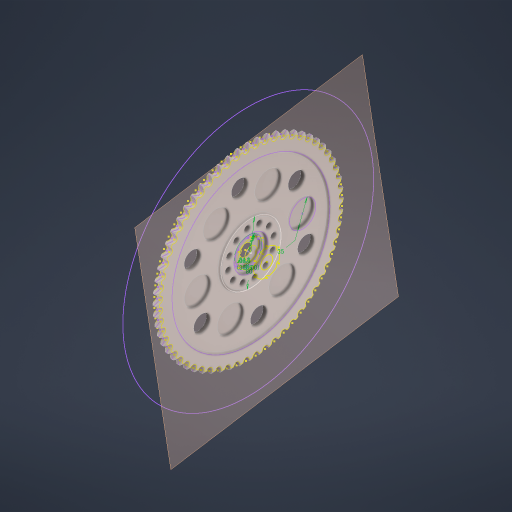
# Autodesk Inventor part: 40A60_()
Saved by Autodesk Inventor 2024.3 (Build 283343000, 343)
## iProperties
Category: PARTsolutions
Company: KANA
Created: 2025-03-03
Part Number: 40A60_()
Material: Generic
Catalog Web Link: www.cadenas.de
Description: 40A-Un-finished
Vendor: KANA
Document SubType Name: Modeling
Designer: psAdmin
Manufacturer: KANA
Mass: 324.137 g
Surface Area: 991.07 cm^2
Volume: 324.137 cm^3
Density: 1 g/cm^3
Appearance: PSOLRGB-175-175-175
PSOL_IDENT_0: {$CADENAS_DATA/23d-libs/kana/sprockets/chain_no_40/un_finished_sprcoket_steel/a_type/40a.prj},156 {V
PSOL_IDENT_1: TYP=3D},{NB=40A60_()},{LINA=40A60},{NN=40A},{DATE=27.06.2023 01:46:20},{GEOMDATE=02.10.2020 05:05:43
PSOL_IDENT_2: },{VERSION=},{LINEID=490},{WBVAR=SURFT},{WBNUMERIC=}  {NB=40A60_()},{LINA=40A60},{KT=DUMMY},{ORDERNO=
PSOL_IDENT_3: 40A60},{TYPE=40A},{NOT=60},{NOTX=60.000},{DP=242.66},{DC=234.71},{DC2=234.71},{DO=250},{T=7.2},{DR=7
PSOL_IDENT_4: .950},{MAT=None},{MATC=},{SD=16},{SURFT=},{SURFTNB=},{DCX2=0},{CAUTION=The tooth profile in the CAD
PSOL_IDENT_5: models differ from the actual shape.}
NB: 40A60_()
NN: 40A
NT: Un-finished
NBSYN: 40A$NOT._($SURFT.)
LINA: 40A60
CATALOG: KANA
TYPE: 40A
NOT: 60
DP: 242.66
DC: 234.71
DC2: 234.71
DO: 250
T: 7.2
SD: 16
SURFT: No symbol : No
CAUTION: The tooth profile in the CAD models differ from the actual shape.
SUPPLIER: KANA
ARTICLENO: 40A60_()
BOMINFO: 40A60
CREATOR: CADENAS GmbH
Title: 40A60
Author: Cadenas PARTsolutions
Comments: Un-finished
Autodesk Inventor part; units mm, degrees
(part 1 of 2)
ref_plane "YZ Plane" through (0, 0, 0) normal (1, 0, 0) x (0, 1, 0)
ref_plane "XZ Plane" through (0, 0, 0) normal (0, 1, 0) x (-1, 0, 0)
ref_plane "XY Plane" through (0, 0, 0) normal (0, 0, 1) x (1, 0, 0)
sketch "Sketch_1" plane through (0, 0, 0) normal (0, 0, 1) x (1, 0, 0)
  line L0 (7.2, 0) -> (0, 0)
  line L1 (0, 8) -> (7.2, 8)
  line L2 (7.2, 8) -> (7.2, 121.6682)
  arc A0 (7.2, 121.6682) -> (5.4, 125) centre (-0.4933, 119.6641) ccw
  line L3 (5.4, 125) -> (1.8, 125)
  arc A1 (1.8, 125) -> (0, 121.6682) centre (7.6933, 119.6641) ccw
  line L4 (0, 121.6682) -> (0, 8)
  constraints: 10 end point, 4 point on circle, 2 centre point
revolve "Revolution1" add sketch "Sketch_1" angle 360 about axis through (7.2, 0, 0) along (1, 0, 0)
sketch "Sketch_2" plane through (3.6, 0, 0) normal (1, 0, 0) x (0, 0, -1)
  circle A0 centre (0, 0) radius 166.6667
  arc A1 (-124.999, 0.5) -> (-124.999, -0.5) centre (0, 0) ccw
  line L0 (-124.999, -0.5) -> (-119.6668, -2.6675)
  arc A2 (-119.2901, -9.8557) -> (-119.6668, -2.6675) centre (-121.1637, -6.3499) ccw
  line L1 (-119.2901, -9.8557) -> (-124.3665, -12.5687)
  arc A3 (-124.3665, -12.5687) -> (-124.262, -13.5632) centre (0, 0) ccw
  line L2 (-124.262, -13.5632) -> (-118.7324, -15.1615)
  arc A4 (-117.6064, -22.2709) -> (-118.7324, -15.1615) centre (-119.8362, -18.9802) ccw
  line L3 (-117.6064, -22.2709) -> (-122.3714, -25.4997)
  arc A5 (-122.3714, -25.4997) -> (-122.1635, -26.4778) centre (0, 0) ccw
  line L4 (-122.1635, -26.4778) -> (-116.4972, -27.4894)
  arc A6 (-114.6342, -34.4421) -> (-116.4972, -27.4894) centre (-117.1958, -31.4025) ccw
  line L5 (-114.6342, -34.4421) -> (-119.0356, -38.1513)
  arc A7 (-119.0356, -38.1513) -> (-118.7266, -39.1023) centre (0, 0) ccw
  line L6 (-118.7266, -39.1023) -> (-112.9856, -39.5161)
  arc A8 (-110.4061, -46.236) -> (-112.9856, -39.5161) centre (-113.2713, -43.4808) ccw
  line L7 (-110.4061, -46.236) -> (-114.3956, -50.3849)
  arc A9 (-114.3956, -50.3849) -> (-113.9889, -51.2984) centre (0, 0) ccw
  line L8 (-113.9889, -51.2984) -> (-108.2361, -51.1098)
  arc A10 (-104.9683, -57.5233) -> (-108.2361, -51.1098) centre (-108.1058, -55.0827) ccw
  line L9 (-104.9683, -57.5233) -> (-108.5023, -62.0665)
  arc A11 (-108.5023, -62.0665) -> (-108.0023, -62.9325) centre (0, 0) ccw
  line L10 (-108.0023, -62.9325) -> (-102.3007, -62.1436)
  arc A12 (-98.3804, -68.1803) -> (-102.3007, -62.1436) centre (-101.7559, -66.0811) ccw
  line L11 (-98.3804, -68.1803) -> (-101.4202, -73.0681)
  arc A13 (-101.4202, -73.0681) -> (-100.8324, -73.8771) centre (0, 0) ccw
  line L12 (-100.8324, -73.8771) -> (-95.2446, -72.4965)
  arc A14 (-90.7147, -78.0904) -> (-95.2446, -72.4965) centre (-94.2911, -76.3554) ccw
  line L13 (-90.7147, -78.0904) -> (-93.2269, -83.2691)
  arc A15 (-93.2269, -83.2691) -> (-92.5578, -84.0122) centre (0, 0) ccw
  line L14 (-92.5578, -84.0122) -> (-87.1448, -82.0551)
  arc A16 (-82.0551, -87.1448) -> (-87.1448, -82.0551) centre (-85.7933, -85.7933) ccw
  line L15 (-82.0551, -87.1448) -> (-84.0122, -92.5578)
  arc A17 (-84.0122, -92.5578) -> (-83.2691, -93.2269) centre (0, 0) ccw
  line L16 (-83.2691, -93.2269) -> (-78.0904, -90.7147)
  arc A18 (-72.4965, -95.2446) -> (-78.0904, -90.7147) centre (-76.3554, -94.2911) ccw
  line L17 (-72.4965, -95.2446) -> (-73.8771, -100.8324)
  arc A19 (-73.8771, -100.8324) -> (-73.0681, -101.4202) centre (0, 0) ccw
  line L18 (-73.0681, -101.4202) -> (-68.1803, -98.3804)
  arc A20 (-62.1436, -102.3007) -> (-68.1803, -98.3804) centre (-66.0811, -101.7559) ccw
  line L19 (-62.1436, -102.3007) -> (-62.9325, -108.0023)
  arc A21 (-62.9325, -108.0023) -> (-62.0665, -108.5023) centre (0, 0) ccw
  line L20 (-62.0665, -108.5023) -> (-57.5233, -104.9683)
  arc A22 (-51.1098, -108.2361) -> (-57.5233, -104.9683) centre (-55.0827, -108.1058) ccw
  line L21 (-51.1098, -108.2361) -> (-51.2984, -113.9889)
  arc A23 (-51.2984, -113.9889) -> (-50.3849, -114.3956) centre (0, 0) ccw
  line L22 (-50.3849, -114.3956) -> (-46.236, -110.4061)
  arc A24 (-39.5161, -112.9856) -> (-46.236, -110.4061) centre (-43.4808, -113.2713) ccw
  line L23 (-39.5161, -112.9856) -> (-39.1023, -118.7266)
  arc A25 (-39.1023, -118.7266) -> (-38.1513, -119.0356) centre (0, 0) ccw
  line L24 (-38.1513, -119.0356) -> (-34.4421, -114.6342)
  arc A26 (-27.4894, -116.4972) -> (-34.4421, -114.6342) centre (-31.4025, -117.1958) ccw
  line L25 (-27.4894, -116.4972) -> (-26.4778, -122.1635)
  arc A27 (-26.4778, -122.1635) -> (-25.4997, -122.3714) centre (0, 0) ccw
  line L26 (-25.4997, -122.3714) -> (-22.2709, -117.6064)
  arc A28 (-15.1615, -118.7324) -> (-22.2709, -117.6064) centre (-18.9802, -119.8362) ccw
  line L27 (-15.1615, -118.7324) -> (-13.5632, -124.262)
  arc A29 (-13.5632, -124.262) -> (-12.5687, -124.3665) centre (0, 0) ccw
  line L28 (-12.5687, -124.3665) -> (-9.8557, -119.2901)
  arc A30 (-2.6675, -119.6668) -> (-9.8557, -119.2901) centre (-6.3499, -121.1637) ccw
  line L29 (-2.6675, -119.6668) -> (-0.5, -124.999)
  arc A31 (-0.5, -124.999) -> (0.5, -124.999) centre (0, 0) ccw
  line L30 (0.5, -124.999) -> (2.6675, -119.6668)
  arc A32 (9.8557, -119.2901) -> (2.6675, -119.6668) centre (6.3499, -121.1637) ccw
  line L31 (9.8557, -119.2901) -> (12.5687, -124.3665)
  arc A33 (12.5687, -124.3665) -> (13.5632, -124.262) centre (0, 0) ccw
  line L32 (13.5632, -124.262) -> (15.1615, -118.7324)
  arc A34 (22.2709, -117.6064) -> (15.1615, -118.7324) centre (18.9802, -119.8362) ccw
  line L33 (22.2709, -117.6064) -> (25.4997, -122.3714)
  arc A35 (25.4997, -122.3714) -> (26.4778, -122.1635) centre (0, 0) ccw
  line L34 (26.4778, -122.1635) -> (27.4894, -116.4972)
  arc A36 (34.4421, -114.6342) -> (27.4894, -116.4972) centre (31.4025, -117.1958) ccw
  line L35 (34.4421, -114.6342) -> (38.1513, -119.0356)
  arc A37 (38.1513, -119.0356) -> (39.1023, -118.7266) centre (0, 0) ccw
  line L36 (39.1023, -118.7266) -> (39.5161, -112.9856)
  arc A38 (46.236, -110.4061) -> (39.5161, -112.9856) centre (43.4808, -113.2713) ccw
  line L37 (46.236, -110.4061) -> (50.3849, -114.3956)
  arc A39 (50.3849, -114.3956) -> (51.2984, -113.9889) centre (0, 0) ccw
  line L38 (51.2984, -113.9889) -> (51.1098, -108.2361)
  arc A40 (57.5233, -104.9683) -> (51.1098, -108.2361) centre (55.0827, -108.1058) ccw
  line L39 (57.5233, -104.9683) -> (62.0665, -108.5023)
  arc A41 (62.0665, -108.5023) -> (62.9325, -108.0023) centre (0, 0) ccw
  line L40 (62.9325, -108.0023) -> (62.1436, -102.3007)
  arc A42 (68.1803, -98.3804) -> (62.1436, -102.3007) centre (66.0811, -101.7559) ccw
  line L41 (68.1803, -98.3804) -> (73.0681, -101.4202)
  arc A43 (73.0681, -101.4202) -> (73.8771, -100.8324) centre (0, 0) ccw
  line L42 (73.8771, -100.8324) -> (72.4965, -95.2446)
  arc A44 (78.0904, -90.7147) -> (72.4965, -95.2446) centre (76.3554, -94.2911) ccw
  line L43 (78.0904, -90.7147) -> (83.2691, -93.2269)
  arc A45 (83.2691, -93.2269) -> (84.0122, -92.5578) centre (0, 0) ccw
  line L44 (84.0122, -92.5578) -> (82.0551, -87.1448)
  arc A46 (87.1448, -82.0551) -> (82.0551, -87.1448) centre (85.7933, -85.7933) ccw
  line L45 (87.1448, -82.0551) -> (92.5578, -84.0122)
  arc A47 (92.5578, -84.0122) -> (93.2269, -83.2691) centre (0, 0) ccw
  line L46 (93.2269, -83.2691) -> (90.7147, -78.0904)
  arc A48 (95.2446, -72.4965) -> (90.7147, -78.0904) centre (94.2911, -76.3554) ccw
  line L47 (95.2446, -72.4965) -> (100.8324, -73.8771)
  arc A49 (100.8324, -73.8771) -> (101.4202, -73.0681) centre (0, 0) ccw
  line L48 (101.4202, -73.0681) -> (98.3804, -68.1803)
  arc A50 (102.3007, -62.1436) -> (98.3804, -68.1803) centre (101.7559, -66.0811) ccw
  line L49 (102.3007, -62.1436) -> (108.0023, -62.9325)
  arc A51 (108.0023, -62.9325) -> (108.5023, -62.0665) centre (0, 0) ccw
  line L50 (108.5023, -62.0665) -> (104.9683, -57.5233)
  arc A52 (108.2361, -51.1098) -> (104.9683, -57.5233) centre (108.1058, -55.0827) ccw
  line L51 (108.2361, -51.1098) -> (113.9889, -51.2984)
  arc A53 (113.9889, -51.2984) -> (114.3956, -50.3849) centre (0, 0) ccw
  line L52 (114.3956, -50.3849) -> (110.4061, -46.236)
  arc A54 (112.9856, -39.5161) -> (110.4061, -46.236) centre (113.2713, -43.4808) ccw
  line L53 (112.9856, -39.5161) -> (118.7266, -39.1023)
  arc A55 (118.7266, -39.1023) -> (119.0356, -38.1513) centre (0, 0) ccw
  line L54 (119.0356, -38.1513) -> (114.6342, -34.4421)
  arc A56 (116.4972, -27.4894) -> (114.6342, -34.4421) centre (117.1958, -31.4025) ccw
  line L55 (116.4972, -27.4894) -> (122.1635, -26.4778)
  arc A57 (122.1635, -26.4778) -> (122.3714, -25.4997) centre (0, 0) ccw
  line L56 (122.3714, -25.4997) -> (117.6064, -22.2709)
  arc A58 (118.7324, -15.1615) -> (117.6064, -22.2709) centre (119.8362, -18.9802) ccw
  line L57 (118.7324, -15.1615) -> (124.262, -13.5632)
  arc A59 (124.262, -13.5632) -> (124.3665, -12.5687) centre (0, 0) ccw
  line L58 (124.3665, -12.5687) -> (119.2901, -9.8557)
  arc A60 (119.6668, -2.6675) -> (119.2901, -9.8557) centre (121.1637, -6.3499) ccw
  line L59 (119.6668, -2.6675) -> (124.999, -0.5)
  arc A61 (124.999, -0.5) -> (124.999, 0.5) centre (0, 0) ccw
  line L60 (124.999, 0.5) -> (119.6668, 2.6675)
  arc A62 (119.2901, 9.8557) -> (119.6668, 2.6675) centre (121.1637, 6.3499) ccw
  line L61 (119.2901, 9.8557) -> (124.3665, 12.5687)
  arc A63 (124.3665, 12.5687) -> (124.262, 13.5632) centre (0, 0) ccw
  line L62 (124.262, 13.5632) -> (118.7324, 15.1615)
  arc A64 (117.6064, 22.2709) -> (118.7324, 15.1615) centre (119.8362, 18.9802) ccw
  line L63 (117.6064, 22.2709) -> (122.3714, 25.4997)
  arc A65 (122.3714, 25.4997) -> (122.1635, 26.4778) centre (0, 0) ccw
  line L64 (122.1635, 26.4778) -> (116.4972, 27.4894)
  arc A66 (114.6342, 34.4421) -> (116.4972, 27.4894) centre (117.1958, 31.4025) ccw
  line L65 (114.6342, 34.4421) -> (119.0356, 38.1513)
  arc A67 (119.0356, 38.1513) -> (118.7266, 39.1023) centre (0, 0) ccw
  line L66 (118.7266, 39.1023) -> (112.9856, 39.5161)
  arc A68 (110.4061, 46.236) -> (112.9856, 39.5161) centre (113.2713, 43.4808) ccw
  line L67 (110.4061, 46.236) -> (114.3956, 50.3849)
  arc A69 (114.3956, 50.3849) -> (113.9889, 51.2984) centre (0, 0) ccw
  line L68 (113.9889, 51.2984) -> (108.2361, 51.1098)
  arc A70 (104.9683, 57.5233) -> (108.2361, 51.1098) centre (108.1058, 55.0827) ccw
  line L69 (104.9683, 57.5233) -> (108.5023, 62.0665)
  arc A71 (108.5023, 62.0665) -> (108.0023, 62.9325) centre (0, 0) ccw
  line L70 (108.0023, 62.9325) -> (102.3007, 62.1436)
  arc A72 (98.3804, 68.1803) -> (102.3007, 62.1436) centre (101.7559, 66.0811) ccw
  line L71 (98.3804, 68.1803) -> (101.4202, 73.0681)
  arc A73 (101.4202, 73.0681) -> (100.8324, 73.8771) centre (0, 0) ccw
  line L72 (100.8324, 73.8771) -> (95.2446, 72.4965)
  arc A74 (90.7147, 78.0904) -> (95.2446, 72.4965) centre (94.2911, 76.3554) ccw
  line L73 (90.7147, 78.0904) -> (93.2269, 83.2691)
  arc A75 (93.2269, 83.2691) -> (92.5578, 84.0122) centre (0, 0) ccw
  line L74 (92.5578, 84.0122) -> (87.1448, 82.0551)
  arc A76 (82.0551, 87.1448) -> (87.1448, 82.0551) centre (85.7933, 85.7933) ccw
  line L75 (82.0551, 87.1448) -> (84.0122, 92.5578)
  arc A77 (84.0122, 92.5578) -> (83.2691, 93.2269) centre (0, 0) ccw
  line L76 (83.2691, 93.2269) -> (78.0904, 90.7147)
  arc A78 (72.4965, 95.2446) -> (78.0904, 90.7147) centre (76.3554, 94.2911) ccw
  line L77 (72.4965, 95.2446) -> (73.8771, 100.8324)
  arc A79 (73.8771, 100.8324) -> (73.0681, 101.4202) centre (0, 0) ccw
  line L78 (73.0681, 101.4202) -> (68.1803, 98.3804)
  arc A80 (62.1436, 102.3007) -> (68.1803, 98.3804) centre (66.0811, 101.7559) ccw
  line L79 (62.1436, 102.3007) -> (62.9325, 108.0023)
  arc A81 (62.9325, 108.0023) -> (62.0665, 108.5023) centre (0, 0) ccw
  line L80 (62.0665, 108.5023) -> (57.5233, 104.9683)
  arc A82 (51.1098, 108.2361) -> (57.5233, 104.9683) centre (55.0827, 108.1058) ccw
  line L81 (51.1098, 108.2361) -> (51.2984, 113.9889)
  arc A83 (51.2984, 113.9889) -> (50.3849, 114.3956) centre (0, 0) ccw
  line L82 (50.3849, 114.3956) -> (46.236, 110.4061)
  arc A84 (39.5161, 112.9856) -> (46.236, 110.4061) centre (43.4808, 113.2713) ccw
  line L83 (39.5161, 112.9856) -> (39.1023, 118.7266)
  arc A85 (39.1023, 118.7266) -> (38.1513, 119.0356) centre (0, 0) ccw
  line L84 (38.1513, 119.0356) -> (34.4421, 114.6342)
  arc A86 (27.4894, 116.4972) -> (34.4421, 114.6342) centre (31.4025, 117.1958) ccw
  line L85 (27.4894, 116.4972) -> (26.4778, 122.1635)
  arc A87 (26.4778, 122.1635) -> (25.4997, 122.3714) centre (0, 0) ccw
  line L86 (25.4997, 122.3714) -> (22.2709, 117.6064)
  arc A88 (15.1615, 118.7324) -> (22.2709, 117.6064) centre (18.9802, 119.8362) ccw
  line L87 (15.1615, 118.7324) -> (13.5632, 124.262)
  arc A89 (13.5632, 124.262) -> (12.5687, 124.3665) centre (0, 0) ccw
  line L88 (12.5687, 124.3665) -> (9.8557, 119.2901)
  arc A90 (2.6675, 119.6668) -> (9.8557, 119.2901) centre (6.3499, 121.1637) ccw
  line L89 (2.6675, 119.6668) -> (0.5, 124.999)
  arc A91 (0.5, 124.999) -> (-0.5, 124.999) centre (0, 0) ccw
  line L90 (-0.5, 124.999) -> (-2.6675, 119.6668)
  arc A92 (-9.8557, 119.2901) -> (-2.6675, 119.6668) centre (-6.3499, 121.1637) ccw
  line L91 (-9.8557, 119.2901) -> (-12.5687, 124.3665)
  arc A93 (-12.5687, 124.3665) -> (-13.5632, 124.262) centre (0, 0) ccw
  line L92 (-13.5632, 124.262) -> (-15.1615, 118.7324)
  arc A94 (-22.2709, 117.6064) -> (-15.1615, 118.7324) centre (-18.9802, 119.8362) ccw
  line L93 (-22.2709, 117.6064) -> (-25.4997, 122.3714)
  arc A95 (-25.4997, 122.3714) -> (-26.4778, 122.1635) centre (0, 0) ccw
  line L94 (-26.4778, 122.1635) -> (-27.4894, 116.4972)
  arc A96 (-34.4421, 114.6342) -> (-27.4894, 116.4972) centre (-31.4025, 117.1958) ccw
  line L95 (-34.4421, 114.6342) -> (-38.1513, 119.0356)
  arc A97 (-38.1513, 119.0356) -> (-39.1023, 118.7266) centre (0, 0) ccw
  line L96 (-39.1023, 118.7266) -> (-39.5161, 112.9856)
  arc A98 (-46.236, 110.4061) -> (-39.5161, 112.9856) centre (-43.4808, 113.2713) ccw
  line L97 (-46.236, 110.4061) -> (-50.3849, 114.3956)
  arc A99 (-50.3849, 114.3956) -> (-51.2984, 113.9889) centre (0, 0) ccw
  line L98 (-51.2984, 113.9889) -> (-51.1098, 108.2361)
  arc A100 (-57.5233, 104.9683) -> (-51.1098, 108.2361) centre (-55.0827, 108.1058) ccw
  line L99 (-57.5233, 104.9683) -> (-62.0665, 108.5023)
  arc A101 (-62.0665, 108.5023) -> (-62.9325, 108.0023) centre (0, 0) ccw
  line L100 (-62.9325, 108.0023) -> (-62.1436, 102.3007)
  arc A102 (-68.1803, 98.3804) -> (-62.1436, 102.3007) centre (-66.0811, 101.7559) ccw
  line L101 (-68.1803, 98.3804) -> (-73.0681, 101.4202)
  arc A103 (-73.0681, 101.4202) -> (-73.8771, 100.8324) centre (0, 0) ccw
  line L102 (-73.8771, 100.8324) -> (-72.4965, 95.2446)
  arc A104 (-78.0904, 90.7147) -> (-72.4965, 95.2446) centre (-76.3554, 94.2911) ccw
  line L103 (-78.0904, 90.7147) -> (-83.2691, 93.2269)
  arc A105 (-83.2691, 93.2269) -> (-84.0122, 92.5578) centre (0, 0) ccw
  line L104 (-84.0122, 92.5578) -> (-82.0551, 87.1448)
  arc A106 (-87.1448, 82.0551) -> (-82.0551, 87.1448) centre (-85.7933, 85.7933) ccw
  line L105 (-87.1448, 82.0551) -> (-92.5578, 84.0122)
  arc A107 (-92.5578, 84.0122) -> (-93.2269, 83.2691) centre (0, 0) ccw
  line L106 (-93.2269, 83.2691) -> (-90.7147, 78.0904)
  arc A108 (-95.2446, 72.4965) -> (-90.7147, 78.0904) centre (-94.2911, 76.3554) ccw
  line L107 (-95.2446, 72.4965) -> (-100.8324, 73.8771)
  arc A109 (-100.8324, 73.8771) -> (-101.4202, 73.0681) centre (0, 0) ccw
  line L108 (-101.4202, 73.0681) -> (-98.3804, 68.1803)
  arc A110 (-102.3007, 62.1436) -> (-98.3804, 68.1803) centre (-101.7559, 66.0811) ccw
  line L109 (-102.3007, 62.1436) -> (-108.0023, 62.9325)
  arc A111 (-108.0023, 62.9325) -> (-108.5023, 62.0665) centre (0, 0) ccw
  line L110 (-108.5023, 62.0665) -> (-104.9683, 57.5233)
  arc A112 (-108.2361, 51.1098) -> (-104.9683, 57.5233) centre (-108.1058, 55.0827) ccw
  line L111 (-108.2361, 51.1098) -> (-113.9889, 51.2984)
  arc A113 (-113.9889, 51.2984) -> (-114.3956, 50.3849) centre (0, 0) ccw
  line L112 (-114.3956, 50.3849) -> (-110.4061, 46.236)
  arc A114 (-112.9856, 39.5161) -> (-110.4061, 46.236) centre (-113.2713, 43.4808) ccw
  line L113 (-112.9856, 39.5161) -> (-118.7266, 39.1023)
  arc A115 (-118.7266, 39.1023) -> (-119.0356, 38.1513) centre (0, 0) ccw
  line L114 (-119.0356, 38.1513) -> (-114.6342, 34.4421)
  arc A116 (-116.4972, 27.4894) -> (-114.6342, 34.4421) centre (-117.1958, 31.4025) ccw
  line L115 (-116.4972, 27.4894) -> (-122.1635, 26.4778)
  arc A117 (-122.1635, 26.4778) -> (-122.3714, 25.4997) centre (0, 0) ccw
  line L116 (-122.3714, 25.4997) -> (-117.6064, 22.2709)
  arc A118 (-118.7324, 15.1615) -> (-117.6064, 22.2709) centre (-119.8362, 18.9802) ccw
  line L117 (-118.7324, 15.1615) -> (-124.262, 13.5632)
  arc A119 (-124.262, 13.5632) -> (-124.3665, 12.5687) centre (0, 0) ccw
  line L118 (-124.3665, 12.5687) -> (-119.2901, 9.8557)
  arc A120 (-119.6668, 2.6675) -> (-119.2901, 9.8557) centre (-121.1637, 6.3499) ccw
  line L119 (-119.6668, 2.6675) -> (-124.999, 0.5)
  circle A121 centre (0, 0) radius 17.4
  line L120 (0, -17.4) -> (0, -15.4)
  line L121 (2.75, -16.847) -> (-2.75, -16.847) construction
  line L122 (-2.75, -16.847) -> (-2.75, -17.953) construction
  line L123 (-2.75, -17.953) -> (2.75, -17.953) construction
  line L124 (2.75, -17.953) -> (2.75, -16.847) construction
  line L125 (2.75, -16.847) -> (-2.75, -17.953) construction
  line L126 (-2.75, -16.847) -> (2.75, -17.953) construction
  arc A122 (2.75, -17.1813) -> (-2.75, -17.1813) centre (0, -18.4134) ccw
  arc A123 (16.2545, -6.2091) -> (13.5045, -10.9722) centre (15.9465, -9.2067) ccw
  arc A124 (13.5045, 10.9722) -> (16.2545, 6.2091) centre (15.9465, 9.2067) ccw
  arc A125 (-2.75, 17.1813) -> (2.75, 17.1813) centre (0, 18.4134) ccw
  arc A126 (-16.2545, 6.2091) -> (-13.5045, 10.9722) centre (-15.9465, 9.2067) ccw
  arc A127 (-13.5045, -10.9722) -> (-16.2545, -6.2091) centre (-15.9465, -9.2067) ccw
  circle A128 centre (0, 0) radius 19.25
  point P0 (13.3368, -7.7)
  point P1 (13.3368, 7.7)
  point P2 (0, 15.4)
  point P3 (-13.3368, 7.7)
  point P4 (-13.3368, -7.7)
  point P5 (16.2545, 6.2091)
  point P6 (13.5045, 10.9722)
  point P7 (-2.75, 17.1813)
  point P8 (-16.2545, 6.2091)
  point P9 (13.5045, -10.9722)
  dimension "d7" = 34.8
  dimension "d8" = 2
  dimension "d9" = 5.5
  dimension "d10" = 360
  dimension "d11" = 38.5
  constraints: 261 point on circle, 254 end point, 129 centre point, 3 coincident, 2 midpoint, 2 parallel, 2 point on line, 1 horizontal, 1 perpendicular, 1 vertical, 31 other
  measures "d7" diameter of A121
  measures "d8" distance of L120.start L120.end
  measures "d9" distance of L124.start L122.end
  measures "d11" diameter of A128
extrude "Extrusion1" cut sketch "Sketch_2" along normal mid plane 7.6 contours A0
ref_plane "Body_XY" through (0, 0, 0) normal (1, 0, 0) x (0, 0, -1)
ref_plane "Body_YZ" through (0, 0, 0) normal (0, 0, -1) x (0, 1, 0)
ref_plane "Body_ZX" through (0, 0, 0) normal (0, 1, 0) x (1, 0, 0)
extrude "押し出し2" cut sketch "Sketch_2" along normal blind 10 contours A121 A123 A122 A127 A126 A125 A124
sketch "スケッチ3" plane through (3.6, 0, 0) normal (1, 0, 0) x (0, 0, -1)
  circle A0 centre (0, 0) radius 8 projected
  arc A1 (13.5045, 10.9722) -> (2.75, 17.1813) centre (0, 0) ccw projected
  arc A2 (-2.75, 17.1813) -> (2.75, 17.1813) centre (0, 18.4134) ccw projected
  arc A3 (-2.75, 17.1813) -> (-13.5045, 10.9722) centre (0, 0) ccw projected
  arc A4 (-16.2545, 6.2091) -> (-13.5045, 10.9722) centre (-15.9465, 9.2067) ccw projected
  arc A5 (-16.2545, 6.2091) -> (-16.2545, -6.2091) centre (0, 0) ccw projected
  arc A6 (-13.5045, -10.9722) -> (-16.2545, -6.2091) centre (-15.9465, -9.2067) ccw projected
  arc A7 (-13.5045, -10.9722) -> (-2.75, -17.1813) centre (0, 0) ccw projected
  arc A8 (2.75, -17.1813) -> (-2.75, -17.1813) centre (0, -18.4134) ccw projected
  arc A9 (2.75, -17.1813) -> (13.5045, -10.9722) centre (0, 0) ccw projected
  arc A10 (16.2545, -6.2091) -> (13.5045, -10.9722) centre (15.9465, -9.2067) ccw projected
  arc A11 (16.2545, -6.2091) -> (16.2545, 6.2091) centre (0, 0) ccw projected
  arc A12 (13.5045, 10.9722) -> (16.2545, 6.2091) centre (15.9465, 9.2067) ccw projected
sketch "スケッチ4" plane through (0, 6.3499, -121.1637) normal (-1, 0, 0) x (0, -0.052336, 0.9986295)
  point P0 (121.33, 0)
extrude "押し出し3" cut sketch "Sketch_2" against normal blind 0.5 contours A121 A123 A122 A127 A126 A125 A124
extrude "押し出し4" cut sketch "スケッチ3" against normal blind 2.75
extrude "押し出し5" cut sketch "Sketch_2" against normal blind 3.5 contours A121 A123 A122 A127 A126 A125 A124
sketch "スケッチ5" plane through (0.1, 0, 0) normal (1, 0, 0) x (0, 0, -1)
  point P0 (0, 0)
sketch "スケッチ6" plane through (0.1, 0, 0) normal (1, 0, 0) x (0, 0, -1)
  circle A0 centre (0, 0) radius 8 projected
  arc A1 (13.5045, 10.9722) -> (2.75, 17.1813) centre (0, 0) ccw projected
  arc A2 (-2.75, 17.1813) -> (2.75, 17.1813) centre (0, 18.4134) ccw projected
  arc A3 (-2.75, 17.1813) -> (-13.5045, 10.9722) centre (0, 0) ccw projected
  arc A4 (-16.2545, 6.2091) -> (-13.5045, 10.9722) centre (-15.9465, 9.2067) ccw projected
  arc A5 (-16.2545, 6.2091) -> (-16.2545, -6.2091) centre (0, 0) ccw projected
  arc A6 (-13.5045, -10.9722) -> (-16.2545, -6.2091) centre (-15.9465, -9.2067) ccw projected
  arc A7 (-13.5045, -10.9722) -> (-2.75, -17.1813) centre (0, 0) ccw projected
  arc A8 (2.75, -17.1813) -> (-2.75, -17.1813) centre (0, -18.4134) ccw projected
  arc A9 (2.75, -17.1813) -> (13.5045, -10.9722) centre (0, 0) ccw projected
  arc A10 (16.2545, -6.2091) -> (13.5045, -10.9722) centre (15.9465, -9.2067) ccw projected
  arc A11 (16.2545, -6.2091) -> (16.2545, 6.2091) centre (0, 0) ccw projected
  arc A12 (13.5045, 10.9722) -> (16.2545, 6.2091) centre (15.9465, 9.2067) ccw projected
ref_plane "作業平面4" through (28.2, 18.9802, -119.8362) normal (1, 0, 0) x (0, 0.1564345, -0.9876883)
sketch "スケッチ7" plane through (28.2, 18.9802, -119.8362) normal (1, 0, 0) x (0, 0.1564345, -0.9876883)
  circle A0 centre (-121.33, 0) radius 8 projected
  arc A1 (-106.2754, 8.7246) -> (-115.9261, 16.5396) centre (-121.33, 0) ccw projected
  arc A2 (-121.3584, 17.4) -> (-115.9261, 16.5396) centre (-118.4495, 18.1867) ccw projected
  arc A3 (-121.3584, 17.4) -> (-132.9518, 12.9497) centre (-121.33, 0) ccw projected
  arc A4 (-136.413, 8.6754) -> (-132.9518, 12.9497) centre (-135.6399, 11.5879) ccw projected
  arc A5 (-136.413, 8.6754) -> (-138.3556, -3.5899) centre (-121.33, 0) ccw projected
  arc A6 (-136.3846, -8.7246) -> (-138.3556, -3.5899) centre (-138.5204, -6.5988) ccw projected
  arc A7 (-136.3846, -8.7246) -> (-126.7339, -16.5396) centre (-121.33, 0) ccw projected
  arc A8 (-121.3016, -17.4) -> (-126.7339, -16.5396) centre (-124.2105, -18.1867) ccw projected
  arc A9 (-121.3016, -17.4) -> (-109.7082, -12.9497) centre (-121.33, 0) ccw projected
  arc A10 (-106.247, -8.6754) -> (-109.7082, -12.9497) centre (-107.0201, -11.5879) ccw projected
  arc A11 (-106.247, -8.6754) -> (-104.3044, 3.5899) centre (-121.33, 0) ccw projected
  arc A12 (-106.2754, 8.7246) -> (-104.3044, 3.5899) centre (-104.1396, 6.5988) ccw projected
sketch "スケッチ8" plane through (7.2, 18.9802, -119.8362) normal (1, 0, 0) x (0, 0.1564345, -0.9876883)
  arc A0 (-106.2754, 8.7246) -> (-104.3044, 3.5899) centre (-104.1396, 6.5988) ccw projected
  arc A1 (-106.247, -8.6754) -> (-104.3044, 3.5899) centre (-121.33, 0) ccw projected
  arc A2 (-106.247, -8.6754) -> (-109.7082, -12.9497) centre (-107.0201, -11.5879) ccw projected
  arc A3 (-121.3016, -17.4) -> (-109.7082, -12.9497) centre (-121.33, 0) ccw projected
  arc A4 (-121.3016, -17.4) -> (-126.7339, -16.5396) centre (-124.2105, -18.1867) ccw projected
  arc A5 (-136.3846, -8.7246) -> (-126.7339, -16.5396) centre (-121.33, 0) ccw projected
  arc A6 (-136.3846, -8.7246) -> (-138.3556, -3.5899) centre (-138.5204, -6.5988) ccw projected
  arc A7 (-136.413, 8.6754) -> (-138.3556, -3.5899) centre (-121.33, 0) ccw projected
  arc A8 (-136.413, 8.6754) -> (-132.9518, 12.9497) centre (-135.6399, 11.5879) ccw projected
  arc A9 (-121.3584, 17.4) -> (-132.9518, 12.9497) centre (-121.33, 0) ccw projected
  arc A10 (-121.3584, 17.4) -> (-115.9261, 16.5396) centre (-118.4495, 18.1867) ccw projected
  arc A11 (-106.2754, 8.7246) -> (-115.9261, 16.5396) centre (-121.33, 0) ccw projected
  line L0 (-1.9668, -8.9268) -> (0.0599, -8.2241) projected
  arc A12 (0.0599, -8.2241) -> (0.2546, -4.5097) centre (-121.33, 0) ccw projected
  line L1 (0.2546, -4.5097) -> (-1.6876, -3.599) projected
  arc A13 (-1.6876, 3.599) -> (-1.6876, -3.599) centre (0, 0) ccw projected
  line L2 (-1.6876, 3.599) -> (0.2546, 4.5097) projected
  arc A14 (0.2546, 4.5097) -> (0.0599, 8.2241) centre (-121.33, 0) ccw projected
  line L3 (0.0599, 8.2241) -> (-1.9668, 8.9268) projected
  arc A15 (-2.7192, 16.0853) -> (-1.9668, 8.9268) centre (-0.6647, 12.6824) ccw projected
  line L4 (-2.7192, 16.0853) -> (-0.8829, 17.194) projected
  arc A16 (-0.8829, 17.194) -> (-1.4648, 20.8677) centre (-121.33, 0) ccw projected
  line L5 (-1.4648, 20.8677) -> (-3.5538, 21.3547) projected
  arc A17 (-5.0503, 28.3954) -> (-3.5538, 21.3547) centre (-2.6514, 25.2259) ccw projected
  line L6 (-5.0503, 28.3954) -> (-3.34, 29.69) projected
  arc A18 (-3.34, 29.69) -> (-4.3027, 33.2828) centre (-121.33, 0) ccw projected
  line L7 (-4.3027, 33.2828) -> (-6.4311, 33.5487) projected
  arc A19 (-8.6554, 40.3944) -> (-6.4311, 33.5487) centre (-5.9383, 37.493) ccw projected
  line L8 (-8.6554, 40.3944) -> (-7.0898, 41.8606) projected
  arc A20 (-7.0898, 41.8606) -> (-8.4227, 45.3331) centre (-121.33, 0) ccw projected
  line L9 (-8.4227, 45.3331) -> (-10.5674, 45.3751) projected
  arc A21 (-13.495, 51.9508) -> (-10.5674, 45.3751) centre (-10.4895, 49.3494) ccw projected
  line L10 (-13.495, 51.9508) -> (-12.0912, 53.5727) projected
  arc A22 (-12.0912, 53.5727) -> (-13.7799, 56.8868) centre (-121.33, 0) ccw projected
  line L11 (-13.7799, 56.8868) -> (-15.9171, 56.7044) projected
  arc A23 (-19.5161, 62.938) -> (-15.9171, 56.7044) centre (-16.2551, 60.665) ccw projected
  line L12 (-19.5161, 62.938) -> (-18.2895, 64.6977) projected
  arc A24 (-18.2895, 64.6977) -> (-20.3153, 67.8172) centre (-121.33, 0) ccw projected
  line L13 (-20.3153, 67.8172) -> (-22.4218, 67.4124) projected
  arc A25 (-26.6527, 73.2357) -> (-22.4218, 67.4124) centre (-23.172, 71.316) ccw projected
  line L14 (-26.6527, 73.2357) -> (-25.6167, 75.114) projected
  arc A26 (-25.6167, 75.114) -> (-27.9575, 78.0046) centre (-121.33, 0) ccw projected
  line L15 (-27.9575, 78.0046) -> (-30.0101, 77.3818) projected
  arc A27 (-34.8265, 82.731) -> (-30.0101, 77.3818) centre (-31.1642, 81.1856) ccw projected
  line L16 (-34.8265, 82.731) -> (-33.9926, 84.7073) projected
  arc A28 (-33.9926, 84.7073) -> (-36.6227, 87.3374) centre (-121.33, 0) ccw projected
  line L17 (-36.6227, 87.3374) -> (-38.599, 86.5035) projected
  arc A29 (-43.9482, 91.3199) -> (-38.599, 86.5035) centre (-40.1444, 90.1658) ccw projected
  line L18 (-43.9482, 91.3199) -> (-43.3254, 93.3725) projected
  arc A30 (-43.3254, 93.3725) -> (-46.216, 95.7133) centre (-121.33, 0) ccw projected
  line L19 (-46.216, 95.7133) -> (-48.0943, 94.6773) projected
  arc A31 (-53.9176, 98.9082) -> (-48.0943, 94.6773) centre (-50.014, 98.158) ccw projected
  line L20 (-53.9176, 98.9082) -> (-53.5128, 101.0147) projected
  arc A32 (-53.5128, 101.0147) -> (-56.6323, 103.0405) centre (-121.33, 0) ccw projected
  line L21 (-56.6323, 103.0405) -> (-58.392, 101.8139) projected
  arc A33 (-64.6256, 105.4129) -> (-58.392, 101.8139) centre (-60.665, 105.0749) ccw projected
  line L22 (-64.6256, 105.4129) -> (-64.4432, 107.5501) projected
  arc A34 (-64.4432, 107.5501) -> (-67.7573, 109.2388) centre (-121.33, 0) ccw projected
  line L23 (-67.7573, 109.2388) -> (-69.3792, 107.835) projected
  arc A35 (-75.9549, 110.7626) -> (-69.3792, 107.835) centre (-71.9806, 110.8405) ccw projected
  line L24 (-75.9549, 110.7626) -> (-75.9969, 112.9073) projected
  arc A36 (-75.9969, 112.9073) -> (-79.4694, 114.2402) centre (-121.33, 0) ccw projected
  line L25 (-79.4694, 114.2402) -> (-80.9356, 112.6746) projected
  arc A37 (-87.7813, 114.8989) -> (-80.9356, 112.6746) centre (-83.837, 115.3917) ccw projected
  line L26 (-87.7813, 114.8989) -> (-88.0472, 117.0273) projected
  arc A38 (-88.0472, 117.0273) -> (-91.64, 117.99) centre (-121.33, 0) ccw projected
  line L27 (-91.64, 117.99) -> (-92.9346, 116.2797) projected
  arc A39 (-99.9753, 117.7762) -> (-92.9346, 116.2797) centre (-96.1041, 118.6786) ccw projected
  line L28 (-99.9753, 117.7762) -> (-100.4623, 119.8652) projected
  arc A40 (-100.4623, 119.8652) -> (-104.136, 120.4471) centre (-121.33, 0) ccw projected
  line L29 (-104.136, 120.4471) -> (-105.2447, 118.6108) projected
  arc A41 (-112.4032, 119.3632) -> (-105.2447, 118.6108) centre (-108.6476, 120.6653) ccw projected
  line L30 (-112.4032, 119.3632) -> (-113.1059, 121.3899) projected
  arc A42 (-113.1059, 121.3899) -> (-116.8203, 121.5846) centre (-121.33, 0) ccw projected
  line L31 (-116.8203, 121.5846) -> (-117.731, 119.6424) projected
  arc A43 (-124.929, 119.6424) -> (-117.731, 119.6424) centre (-121.33, 121.33) ccw projected
  line L32 (-124.929, 119.6424) -> (-125.8397, 121.5846) projected
  arc A44 (-125.8397, 121.5846) -> (-129.5541, 121.3899) centre (-121.33, 0) ccw projected
  line L33 (-129.5541, 121.3899) -> (-130.2568, 119.3632) projected
  arc A45 (-137.4153, 118.6108) -> (-130.2568, 119.3632) centre (-134.0124, 120.6653) ccw projected
  line L34 (-137.4153, 118.6108) -> (-138.524, 120.4471) projected
  arc A46 (-138.524, 120.4471) -> (-142.1977, 119.8652) centre (-121.33, 0) ccw projected
  line L35 (-142.1977, 119.8652) -> (-142.6847, 117.7762) projected
  arc A47 (-149.7254, 116.2797) -> (-142.6847, 117.7762) centre (-146.5559, 118.6786) ccw projected
  line L36 (-149.7254, 116.2797) -> (-151.02, 117.99) projected
  arc A48 (-151.02, 117.99) -> (-154.6128, 117.0273) centre (-121.33, 0) ccw projected
  line L37 (-154.6128, 117.0273) -> (-154.8787, 114.8989) projected
  arc A49 (-161.7244, 112.6746) -> (-154.8787, 114.8989) centre (-158.823, 115.3917) ccw projected
  line L38 (-161.7244, 112.6746) -> (-163.1906, 114.2402) projected
  arc A50 (-163.1906, 114.2402) -> (-166.6631, 112.9073) centre (-121.33, 0) ccw projected
  line L39 (-166.6631, 112.9073) -> (-166.7051, 110.7626) projected
  arc A51 (-173.2808, 107.835) -> (-166.7051, 110.7626) centre (-170.6794, 110.8405) ccw projected
  line L40 (-173.2808, 107.835) -> (-174.9027, 109.2388) projected
  arc A52 (-174.9027, 109.2388) -> (-178.2168, 107.5501) centre (-121.33, 0) ccw projected
  line L41 (-178.2168, 107.5501) -> (-178.0344, 105.4129) projected
  arc A53 (-184.268, 101.8139) -> (-178.0344, 105.4129) centre (-181.995, 105.0749) ccw projected
  line L42 (-184.268, 101.8139) -> (-186.0277, 103.0405) projected
  arc A54 (-186.0277, 103.0405) -> (-189.1472, 101.0147) centre (-121.33, 0) ccw projected
  line L43 (-189.1472, 101.0147) -> (-188.7424, 98.9082) projected
  arc A55 (-194.5657, 94.6773) -> (-188.7424, 98.9082) centre (-192.646, 98.158) ccw projected
  line L44 (-194.5657, 94.6773) -> (-196.444, 95.7133) projected
  arc A56 (-196.444, 95.7133) -> (-199.3346, 93.3725) centre (-121.33, 0) ccw projected
  line L45 (-199.3346, 93.3725) -> (-198.7118, 91.3199) projected
  arc A57 (-204.061, 86.5035) -> (-198.7118, 91.3199) centre (-202.5156, 90.1658) ccw projected
  line L46 (-204.061, 86.5035) -> (-206.0373, 87.3374) projected
  arc A58 (-206.0373, 87.3374) -> (-208.6674, 84.7073) centre (-121.33, 0) ccw projected
  line L47 (-208.6674, 84.7073) -> (-207.8335, 82.731) projected
  arc A59 (-212.6499, 77.3818) -> (-207.8335, 82.731) centre (-211.4958, 81.1856) ccw projected
  line L48 (-212.6499, 77.3818) -> (-214.7025, 78.0046) projected
  arc A60 (-214.7025, 78.0046) -> (-217.0433, 75.114) centre (-121.33, 0) ccw projected
  line L49 (-217.0433, 75.114) -> (-216.0073, 73.2357) projected
  arc A61 (-220.2382, 67.4124) -> (-216.0073, 73.2357) centre (-219.488, 71.316) ccw projected
  line L50 (-220.2382, 67.4124) -> (-222.3447, 67.8172) projected
  arc A62 (-222.3447, 67.8172) -> (-224.3705, 64.6977) centre (-121.33, 0) ccw projected
  line L51 (-224.3705, 64.6977) -> (-223.1439, 62.938) projected
  arc A63 (-226.7429, 56.7044) -> (-223.1439, 62.938) centre (-226.4049, 60.665) ccw projected
  line L52 (-226.7429, 56.7044) -> (-228.8801, 56.8868) projected
  arc A64 (-228.8801, 56.8868) -> (-230.5688, 53.5727) centre (-121.33, 0) ccw projected
  line L53 (-230.5688, 53.5727) -> (-229.165, 51.9508) projected
  arc A65 (-232.0926, 45.3751) -> (-229.165, 51.9508) centre (-232.1705, 49.3494) ccw projected
  line L54 (-232.0926, 45.3751) -> (-234.2373, 45.3331) projected
  arc A66 (-234.2373, 45.3331) -> (-235.5702, 41.8606) centre (-121.33, 0) ccw projected
  line L55 (-235.5702, 41.8606) -> (-234.0046, 40.3944) projected
  arc A67 (-236.2289, 33.5487) -> (-234.0046, 40.3944) centre (-236.7217, 37.493) ccw projected
  line L56 (-236.2289, 33.5487) -> (-238.3573, 33.2828) projected
  arc A68 (-238.3573, 33.2828) -> (-239.32, 29.69) centre (-121.33, 0) ccw projected
  line L57 (-239.32, 29.69) -> (-237.6097, 28.3954) projected
  arc A69 (-239.1062, 21.3547) -> (-237.6097, 28.3954) centre (-240.0086, 25.2259) ccw projected
  line L58 (-239.1062, 21.3547) -> (-241.1952, 20.8677) projected
  arc A70 (-241.1952, 20.8677) -> (-241.7771, 17.194) centre (-121.33, 0) ccw projected
  line L59 (-241.7771, 17.194) -> (-239.9408, 16.0853) projected
  arc A71 (-240.6932, 8.9268) -> (-239.9408, 16.0853) centre (-241.9953, 12.6824) ccw projected
  line L60 (-240.6932, 8.9268) -> (-242.7199, 8.2241) projected
  arc A72 (-242.7199, 8.2241) -> (-242.9146, 4.5097) centre (-121.33, 0) ccw projected
  line L61 (-242.9146, 4.5097) -> (-240.9724, 3.599) projected
  arc A73 (-240.9724, -3.599) -> (-240.9724, 3.599) centre (-242.66, 0) ccw projected
  line L62 (-240.9724, -3.599) -> (-242.9146, -4.5097) projected
  arc A74 (-242.9146, -4.5097) -> (-242.7199, -8.2241) centre (-121.33, 0) ccw projected
  line L63 (-242.7199, -8.2241) -> (-240.6932, -8.9268) projected
  arc A75 (-239.9408, -16.0853) -> (-240.6932, -8.9268) centre (-241.9953, -12.6824) ccw projected
  line L64 (-239.9408, -16.0853) -> (-241.7771, -17.194) projected
  arc A76 (-241.7771, -17.194) -> (-241.1952, -20.8677) centre (-121.33, 0) ccw projected
  line L65 (-241.1952, -20.8677) -> (-239.1062, -21.3547) projected
  arc A77 (-237.6097, -28.3954) -> (-239.1062, -21.3547) centre (-240.0086, -25.2259) ccw projected
  line L66 (-237.6097, -28.3954) -> (-239.32, -29.69) projected
  arc A78 (-239.32, -29.69) -> (-238.3573, -33.2828) centre (-121.33, 0) ccw projected
  line L67 (-238.3573, -33.2828) -> (-236.2289, -33.5487) projected
  arc A79 (-234.0046, -40.3944) -> (-236.2289, -33.5487) centre (-236.7217, -37.493) ccw projected
  line L68 (-234.0046, -40.3944) -> (-235.5702, -41.8606) projected
  arc A80 (-235.5702, -41.8606) -> (-234.2373, -45.3331) centre (-121.33, 0) ccw projected
  line L69 (-234.2373, -45.3331) -> (-232.0926, -45.3751) projected
  arc A81 (-229.165, -51.9508) -> (-232.0926, -45.3751) centre (-232.1705, -49.3494) ccw projected
  line L70 (-229.165, -51.9508) -> (-230.5688, -53.5727) projected
  arc A82 (-230.5688, -53.5727) -> (-228.8801, -56.8868) centre (-121.33, 0) ccw projected
  line L71 (-228.8801, -56.8868) -> (-226.7429, -56.7044) projected
  arc A83 (-223.1439, -62.938) -> (-226.7429, -56.7044) centre (-226.4049, -60.665) ccw projected
  line L72 (-223.1439, -62.938) -> (-224.3705, -64.6977) projected
  arc A84 (-224.3705, -64.6977) -> (-222.3447, -67.8172) centre (-121.33, 0) ccw projected
  line L73 (-222.3447, -67.8172) -> (-220.2382, -67.4124) projected
  arc A85 (-216.0073, -73.2357) -> (-220.2382, -67.4124) centre (-219.488, -71.316) ccw projected
  line L74 (-216.0073, -73.2357) -> (-217.0433, -75.114) projected
  arc A86 (-217.0433, -75.114) -> (-214.7025, -78.0046) centre (-121.33, 0) ccw projected
  line L75 (-214.7025, -78.0046) -> (-212.6499, -77.3818) projected
  arc A87 (-207.8335, -82.731) -> (-212.6499, -77.3818) centre (-211.4958, -81.1856) ccw projected
  line L76 (-207.8335, -82.731) -> (-208.6674, -84.7073) projected
  arc A88 (-208.6674, -84.7073) -> (-206.0373, -87.3374) centre (-121.33, 0) ccw projected
  line L77 (-206.0373, -87.3374) -> (-204.061, -86.5035) projected
  arc A89 (-198.7118, -91.3199) -> (-204.061, -86.5035) centre (-202.5156, -90.1658) ccw projected
  line L78 (-198.7118, -91.3199) -> (-199.3346, -93.3725) projected
  arc A90 (-199.3346, -93.3725) -> (-196.444, -95.7133) centre (-121.33, 0) ccw projected
  line L79 (-196.444, -95.7133) -> (-194.5657, -94.6773) projected
  arc A91 (-188.7424, -98.9082) -> (-194.5657, -94.6773) centre (-192.646, -98.158) ccw projected
  line L80 (-188.7424, -98.9082) -> (-189.1472, -101.0147) projected
  arc A92 (-189.1472, -101.0147) -> (-186.0277, -103.0405) centre (-121.33, 0) ccw projected
  line L81 (-186.0277, -103.0405) -> (-184.268, -101.8139) projected
  arc A93 (-178.0344, -105.4129) -> (-184.268, -101.8139) centre (-181.995, -105.0749) ccw projected
  line L82 (-178.0344, -105.4129) -> (-178.2168, -107.5501) projected
  arc A94 (-178.2168, -107.5501) -> (-174.9027, -109.2388) centre (-121.33, 0) ccw projected
  line L83 (-174.9027, -109.2388) -> (-173.2808, -107.835) projected
  arc A95 (-166.7051, -110.7626) -> (-173.2808, -107.835) centre (-170.6794, -110.8405) ccw projected
  line L84 (-166.7051, -110.7626) -> (-166.6631, -112.9073) projected
  arc A96 (-166.6631, -112.9073) -> (-163.1906, -114.2402) centre (-121.33, 0) ccw projected
  line L85 (-163.1906, -114.2402) -> (-161.7244, -112.6746) projected
  arc A97 (-154.8787, -114.8989) -> (-161.7244, -112.6746) centre (-158.823, -115.3917) ccw projected
  line L86 (-154.8787, -114.8989) -> (-154.6128, -117.0273) projected
  arc A98 (-154.6128, -117.0273) -> (-151.02, -117.99) centre (-121.33, 0) ccw projected
  line L87 (-151.02, -117.99) -> (-149.7254, -116.2797) projected
  arc A99 (-142.6847, -117.7762) -> (-149.7254, -116.2797) centre (-146.5559, -118.6786) ccw projected
  line L88 (-142.6847, -117.7762) -> (-142.1977, -119.8652) projected
  arc A100 (-142.1977, -119.8652) -> (-138.524, -120.4471) centre (-121.33, 0) ccw projected
  line L89 (-138.524, -120.4471) -> (-137.4153, -118.6108) projected
  arc A101 (-130.2568, -119.3632) -> (-137.4153, -118.6108) centre (-134.0124, -120.6653) ccw projected
  line L90 (-130.2568, -119.3632) -> (-129.5541, -121.3899) projected
  arc A102 (-129.5541, -121.3899) -> (-125.8397, -121.5846) centre (-121.33, 0) ccw projected
  line L91 (-125.8397, -121.5846) -> (-124.929, -119.6424) projected
  arc A103 (-117.731, -119.6424) -> (-124.929, -119.6424) centre (-121.33, -121.33) ccw projected
  line L92 (-117.731, -119.6424) -> (-116.8203, -121.5846) projected
  arc A104 (-116.8203, -121.5846) -> (-113.1059, -121.3899) centre (-121.33, 0) ccw projected
  line L93 (-113.1059, -121.3899) -> (-112.4032, -119.3632) projected
  arc A105 (-105.2447, -118.6108) -> (-112.4032, -119.3632) centre (-108.6476, -120.6653) ccw projected
  line L94 (-105.2447, -118.6108) -> (-104.136, -120.4471) projected
  arc A106 (-104.136, -120.4471) -> (-100.4623, -119.8652) centre (-121.33, 0) ccw projected
  line L95 (-100.4623, -119.8652) -> (-99.9753, -117.7762) projected
  arc A107 (-92.9346, -116.2797) -> (-99.9753, -117.7762) centre (-96.1041, -118.6786) ccw projected
  line L96 (-92.9346, -116.2797) -> (-91.64, -117.99) projected
  arc A108 (-91.64, -117.99) -> (-88.0472, -117.0273) centre (-121.33, 0) ccw projected
  line L97 (-88.0472, -117.0273) -> (-87.7813, -114.8989) projected
  arc A109 (-80.9356, -112.6746) -> (-87.7813, -114.8989) centre (-83.837, -115.3917) ccw projected
  line L98 (-80.9356, -112.6746) -> (-79.4694, -114.2402) projected
  arc A110 (-79.4694, -114.2402) -> (-75.9969, -112.9073) centre (-121.33, 0) ccw projected
  line L99 (-75.9969, -112.9073) -> (-75.9549, -110.7626) projected
  arc A111 (-69.3792, -107.835) -> (-75.9549, -110.7626) centre (-71.9806, -110.8405) ccw projected
  line L100 (-69.3792, -107.835) -> (-67.7573, -109.2388) projected
  arc A112 (-67.7573, -109.2388) -> (-64.4432, -107.5501) centre (-121.33, 0) ccw projected
  line L101 (-64.4432, -107.5501) -> (-64.6256, -105.4129) projected
  arc A113 (-58.392, -101.8139) -> (-64.6256, -105.4129) centre (-60.665, -105.0749) ccw projected
  line L102 (-58.392, -101.8139) -> (-56.6323, -103.0405) projected
  arc A114 (-56.6323, -103.0405) -> (-53.5128, -101.0147) centre (-121.33, 0) ccw projected
  line L103 (-53.5128, -101.0147) -> (-53.9176, -98.9082) projected
  arc A115 (-48.0943, -94.6773) -> (-53.9176, -98.9082) centre (-50.014, -98.158) ccw projected
  line L104 (-48.0943, -94.6773) -> (-46.216, -95.7133) projected
  arc A116 (-46.216, -95.7133) -> (-43.3254, -93.3725) centre (-121.33, 0) ccw projected
  line L105 (-43.3254, -93.3725) -> (-43.9482, -91.3199) projected
  arc A117 (-38.599, -86.5035) -> (-43.9482, -91.3199) centre (-40.1444, -90.1658) ccw projected
  line L106 (-38.599, -86.5035) -> (-36.6227, -87.3374) projected
  arc A118 (-36.6227, -87.3374) -> (-33.9926, -84.7073) centre (-121.33, 0) ccw projected
  line L107 (-33.9926, -84.7073) -> (-34.8265, -82.731) projected
  arc A119 (-30.0101, -77.3818) -> (-34.8265, -82.731) centre (-31.1642, -81.1856) ccw projected
  line L108 (-30.0101, -77.3818) -> (-27.9575, -78.0046) projected
  arc A120 (-27.9575, -78.0046) -> (-25.6167, -75.114) centre (-121.33, 0) ccw projected
  line L109 (-25.6167, -75.114) -> (-26.6527, -73.2357) projected
  arc A121 (-22.4218, -67.4124) -> (-26.6527, -73.2357) centre (-23.172, -71.316) ccw projected
  line L110 (-22.4218, -67.4124) -> (-20.3153, -67.8172) projected
  arc A122 (-20.3153, -67.8172) -> (-18.2895, -64.6977) centre (-121.33, 0) ccw projected
  line L111 (-18.2895, -64.6977) -> (-19.5161, -62.938) projected
  arc A123 (-15.9171, -56.7044) -> (-19.5161, -62.938) centre (-16.2551, -60.665) ccw projected
  line L112 (-15.9171, -56.7044) -> (-13.7799, -56.8868) projected
  arc A124 (-13.7799, -56.8868) -> (-12.0912, -53.5727) centre (-121.33, 0) ccw projected
  line L113 (-12.0912, -53.5727) -> (-13.495, -51.9508) projected
  arc A125 (-10.5674, -45.3751) -> (-13.495, -51.9508) centre (-10.4895, -49.3494) ccw projected
  line L114 (-10.5674, -45.3751) -> (-8.4227, -45.3331) projected
  arc A126 (-8.4227, -45.3331) -> (-7.0898, -41.8606) centre (-121.33, 0) ccw projected
  line L115 (-7.0898, -41.8606) -> (-8.6554, -40.3944) projected
  arc A127 (-6.4311, -33.5487) -> (-8.6554, -40.3944) centre (-5.9383, -37.493) ccw projected
  line L116 (-6.4311, -33.5487) -> (-4.3027, -33.2828) projected
  arc A128 (-4.3027, -33.2828) -> (-3.34, -29.69) centre (-121.33, 0) ccw projected
  line L117 (-3.34, -29.69) -> (-5.0503, -28.3954) projected
  arc A129 (-3.5538, -21.3547) -> (-5.0503, -28.3954) centre (-2.6514, -25.2259) ccw projected
  line L118 (-3.5538, -21.3547) -> (-1.4648, -20.8677) projected
  arc A130 (-1.4648, -20.8677) -> (-0.8829, -17.194) centre (-121.33, 0) ccw projected
  line L119 (-0.8829, -17.194) -> (-2.7192, -16.0853) projected
  arc A131 (-1.9668, -8.9268) -> (-2.7192, -16.0853) centre (-0.6647, -12.6824) ccw projected
  circle A132 centre (-121.33, 0) radius 8 projected
  arc A133 (-106.2754, 8.7246) -> (-115.9261, 16.5396) centre (-121.33, 0) ccw projected
  arc A134 (-121.3584, 17.4) -> (-115.9261, 16.5396) centre (-118.4495, 18.1867) ccw projected
  arc A135 (-121.3584, 17.4) -> (-132.9518, 12.9497) centre (-121.33, 0) ccw projected
  arc A136 (-136.413, 8.6754) -> (-132.9518, 12.9497) centre (-135.6399, 11.5879) ccw projected
  arc A137 (-136.413, 8.6754) -> (-138.3556, -3.5899) centre (-121.33, 0) ccw projected
  arc A138 (-136.3846, -8.7246) -> (-138.3556, -3.5899) centre (-138.5204, -6.5988) ccw projected
  arc A139 (-136.3846, -8.7246) -> (-126.7339, -16.5396) centre (-121.33, 0) ccw projected
  arc A140 (-121.3016, -17.4) -> (-126.7339, -16.5396) centre (-124.2105, -18.1867) ccw projected
  arc A141 (-121.3016, -17.4) -> (-109.7082, -12.9497) centre (-121.33, 0) ccw projected
  arc A142 (-106.247, -8.6754) -> (-109.7082, -12.9497) centre (-107.0201, -11.5879) ccw projected
  arc A143 (-106.247, -8.6754) -> (-104.3044, 3.5899) centre (-121.33, 0) ccw projected
  arc A144 (-106.2754, 8.7246) -> (-104.3044, 3.5899) centre (-104.1396, 6.5988) ccw projected
  circle A145 centre (-121.33, 0) radius 22.643
  circle A146 centre (-121.33, 0) radius 104.8596
  circle A147 centre (-121.33, 0) radius 40
  circle A148 centre (-51.7888, 0) radius 17.5
  dimension "d23" = 80
  dimension "d26" = 35
  constraints: 4 centre point, 3 coincident
  measures "d23" diameter of A147
  measures "d26" diameter of A148
extrude "押し出し6" cut sketch "スケッチ8" against normal blind 4.7 contours A145
extrude "押し出し7" cut sketch "スケッチ8" against normal blind 2.2 contours A146 | A148
extrude "押し出し8" cut sketch "スケッチ8" against normal blind 6.2 contours A148